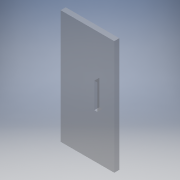
# Autodesk Inventor part: Front_wall
Saved by Autodesk Inventor 2016 (Build 200138000, 138)
## iProperties
Created: 2015-06-25
Part Number: Front_wall
Material: Generic
Document SubType Name: Modeling
Designer: Openlab
Density: 1 g/cm^3
Appearance: Polycarbonate - Clear
Author: Openlab
Autodesk Inventor part; units mm, degrees
ref_plane "YZ Plane" through (0, 0, 0) normal (1, 0, 0) x (0, 1, 0)
ref_plane "XZ Plane" through (0, 0, 0) normal (0, 1, 0) x (-1, 0, 0)
ref_plane "XY Plane" through (0, 0, 0) normal (0, 0, 1) x (1, 0, 0)
sketch "Sketch1" plane through (0, 0, 0) normal (0, 1, 0) x (-1, 0, 0)
  line L0 (15.9236, -19.9274) -> (15.9236, -42.3236) construction
  line L1 (13.2323, -33.5) -> (6.4845, -33.5) construction
  line L2 (31.5, -67) -> (31.5, 0)
  line L3 (0, 0) -> (0, -67)
  line L4 (31.5, 0) -> (0, 0)
  line L5 (0, -67) -> (31.5, -67)
  line L6 (11.7234, -41) -> (9.9234, -41)
  line L7 (9.9234, -41) -> (9.9234, -26)
  line L8 (9.9234, -26) -> (11.7234, -26)
  line L9 (11.7234, -26) -> (11.7234, -41)
  line L10 (26.5, -3) -> (19.5, -3)
  line L11 (19.5, -3) -> (19.5, -6)
  line L12 (19.5, -6) -> (26.5, -6)
  line L13 (26.5, -6) -> (26.5, -3)
  line L14 (12.3471, -3) -> (5.3471, -3)
  line L15 (5.3471, -3) -> (5.3471, -6)
  line L16 (5.3471, -6) -> (12.3471, -6)
  line L17 (12.3471, -6) -> (12.3471, -3)
  line L18 (26.5, -61) -> (19.5, -61)
  line L19 (19.5, -61) -> (19.5, -64)
  line L20 (19.5, -64) -> (26.5, -64)
  line L21 (26.5, -64) -> (26.5, -61)
  line L22 (12.3471, -61) -> (5.3471, -61)
  line L23 (5.3471, -61) -> (5.3471, -64)
  line L24 (5.3471, -64) -> (12.3471, -64)
  line L25 (12.3471, -64) -> (12.3471, -61)
  dimension "d22" = 15
  dimension "d24" = 1.8
  dimension "d25" = 31.5
  dimension "d26" = 67
  dimension "d27" = 7
  dimension "d28" = 3
  dimension "d29" = 5
  dimension "d30" = 3
  constraints: 52 end point, 12 parallel, 7 horizontal, 7 point on line, 6 perpendicular, 3 equal length, 1 coincident, 1 vertical, 4 other
  measures "d22" distance of L8.end L6.start
  measures "d24" distance of L7.end L8.end
  measures "d25" distance of L2.end L3.start
  measures "d26" distance of L2.start L2.end
  measures "d27" distance of L11.end L12.end
  measures "d28" distance of L14.end L15.end
  measures "d29" distance between parallel lines of L13 L2
  measures "d30" distance between parallel lines of L5 L24
extrude "Extrusion1" add sketch "Sketch1" along normal blind 3 contours L5 L3 L4 L2 | L13 L12 L11 L10 | L17 L16 L15 L14 | L21 L20 L19 L18 | L25 L24 L23 L22
body "Solid1"
